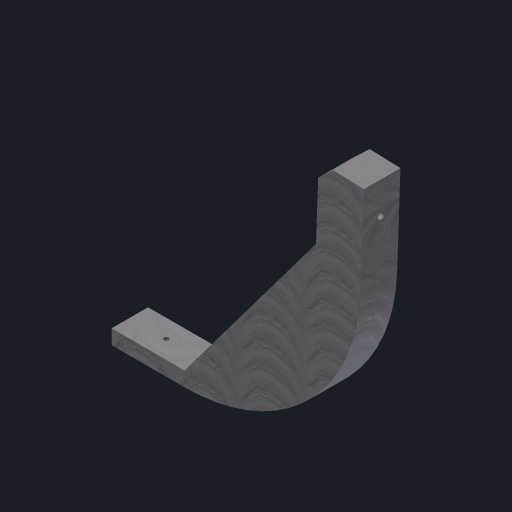
# Autodesk Inventor part: ESQUINA_REDONDEADA_TRASERA
Saved by Autodesk Inventor 2024.3 (Build 283343000, 343)
## iProperties
Created: 2024-06-30
Part Number: ESQUINA_REDONDEADA_TRASERA
Material: Steel, Mild, Welded
Document SubType Name: Modeling
Designer: Niler
Density: 7.85 g/cm^3
Appearance: Weld - Steel Mild
Author: Niler
Autodesk Inventor part; units mm, degrees
ref_plane "YZ Plane" through (0, 0, 0) normal (1, 0, 0) x (0, 1, 0)
ref_plane "XZ Plane" through (0, 0, 0) normal (0, 1, 0) x (-1, 0, 0)
ref_plane "XY Plane" through (0, 0, 0) normal (0, 0, 1) x (1, 0, 0)
sketch "Sketch1" plane through (0, 0, 0) normal (0, 0, 1) x (1, 0, 0)
  line L0 (0, 0) -> (50, 0)
  line L1 (50, 0) -> (140.0002, 119.9998)
  line L2 (140.0002, 119.9998) -> (141.8074, 169.9998)
  line L3 (172.7872, 168.8801) -> (170.5233, 106.2458)
  line L4 (0, -10) -> (50, -10)
  arc A0 (50, -10) -> (170.5233, 106.2458) centre (50, 110.602) ccw
  line L5 (0, -10) -> (0, 0)
  line L6 (141.8074, 169.9998) -> (172.7872, 168.8801)
  line L7 (140.0002, 119.9998) -> (171.0205, 119.9998)
  dimension "d0" = 150
  dimension "d1" = 126.87
  dimension "d2" = 50
  dimension "d3" = 145.2
  dimension "d4" = 31
  dimension "d5" = 10
  dimension "d6" = 50
  constraints: 16 end point, 3 horizontal, 2 parallel, 2 point on circle, 2 tangent, 1 centre point, 1 perpendicular, 1 point on line, 1 vertical, 1 vertical alignment
  measures "d0" distance of L0.end L1.end
  measures "d1" angle of L0 L1
  measures "d2" distance of L0.start L0.end
  measures "d3" angle of L2 L1
  measures "d4" distance between parallel lines of L2 L3
  measures "d5" distance between parallel lines of L0 L4
  measures "d6" vertical distance of L1.end L2.end
extrude "Extrusion1" add sketch "Sketch1" along normal blind 25
sketch "Sketch2" plane through (0, -10, 0) normal (0, -1, 0) x (1, 0, 0)
  line L0 (0, 0) -> (50, 0) projected
  line L1 (50, 0) -> (50, 25) projected
  line L2 (0, 25) -> (50, 25) projected
  line L3 (0, 0) -> (0, 25) projected
  circle A0 centre (25, 12.5) radius 1.65
  point P0 (50, 12.5)
  point P1 (25, 25)
  dimension "d9" = 3.3
  constraints: 2 midpoint, 1 centre point, 1 horizontal alignment, 1 vertical alignment
  measures "d9" diameter of A0
extrude "Extrusion2" cut sketch "Sketch2" against normal through all contours A0
sketch "Sketch3" plane through (172.7872, 168.8801, 25) normal (0.9993474, -0.0361205, 0) x (0, 0, -1)
  line L0 (25, -62.6752) -> (25, 0) projected
  line L1 (25, 0) -> (0, 0) projected
  line L2 (0, -62.6752) -> (0, 0) projected
  line L3 (25, -62.6752) -> (0, -62.6752) projected
  circle A0 centre (12.5, -22.6752) radius 2.15
  point P0 (25, -175.0111)
  point P1 (12.5, -62.6752)
  dimension "d12" = 4.3
  dimension "d13" = 40
  constraints: 1 centre point, 1 midpoint, 1 vertical alignment
  measures "d12" diameter of A0
  measures "d13" distance from line of L3 A0.centre
extrude "Extrusion3" cut sketch "Sketch3" against normal through all contours A0
chamfer "Chamfer1" distance 10 angle 45 1 edges at (141.8074, 169.9998, 12.5)
body "Solid1"
